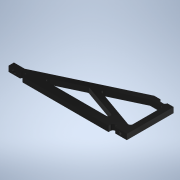
# Autodesk Inventor part: ForeArm_diagonal
Saved by Autodesk Inventor 2020.4 (Build 244396000, 396)
## iProperties
Created: 2016-05-04
Part Number: ForeArm_diagonal
Material: アセタール樹脂、黒
Document SubType Name: Modeling
Designer: hiroaki
Density: 1.425 g/cm^3
Appearance: 滑らか - 黒
Mass: 16.6114 g
Surface Area: 81.8888 cm^2
Volume: 11.6571 cm^3
Description: POM T5
Author: hiroaki
Autodesk Inventor part; units mm, degrees
ref_plane "YZ Plane" through (0, 0, 0) normal (1, 0, 0) x (0, 1, 0)
ref_plane "XZ Plane" through (0, 0, 0) normal (0, 1, 0) x (-1, 0, 0)
ref_plane "XY Plane" through (0, 0, 0) normal (0, 0, 1) x (1, 0, 0)
sketch "スケッチ1" plane through (0, 0, 0) normal (0, 0, 1) x (1, 0, 0)
  line L0 (-55, -21.75) -> (55, -21.75) construction
  line L1 (55, -21.75) -> (55, 21.75) construction
  line L2 (55, 21.75) -> (-55, 21.75) construction
  line L3 (-55, 21.75) -> (-55, -21.75) construction
  line L4 (-55, -21.75) -> (55, 21.75) construction
  line L5 (55, -21.75) -> (-55, 21.75) construction
  line L6 (-50, 21.75) -> (-50, -21.75) construction
  line L7 (0, 0) -> (0, 21.75) construction
  line L8 (0, 0) -> (-55, 0) construction
  line L9 (50, 21.75) -> (50, -11.2747) construction
  line L10 (-55, -21.75) -> (-44.2, -21.75)
  line L11 (47, 21.75) -> (47, 23.75)
  line L12 (47, 23.75) -> (45, 23.75)
  line L13 (45, 23.75) -> (45, 21.75)
  line L14 (49.2, 21.75) -> (55, 21.75)
  line L15 (55, 21.75) -> (55, -21.75)
  line L16 (55, -21.75) -> (44.2, -21.75)
  line L17 (-40, -21.75) -> (-40, -23.75)
  line L18 (-40, -23.75) -> (40, -23.75)
  line L19 (40, -23.75) -> (40, -21.75)
  arc A0 (42.8, 21.75) -> (47, 21.75) centre (44.9, 21.75) ccw
  arc A1 (45, 21.75) -> (49.2, 21.75) centre (47.1, 21.75) ccw
  arc A2 (-40, -21.75) -> (-44.2, -21.75) centre (-42.1, -21.75) ccw
  arc A3 (44.2, -21.75) -> (40, -21.75) centre (42.1, -21.75) ccw
  line L20 (-55, -21.75) -> (-55, -16.75)
  line L21 (42.8, 21.75) -> (37, 21.75)
  line L22 (49.45, 24.476) -> (52.55, 24.476) construction
  line L23 (52.55, 24.476) -> (52.55, 13.3235) construction
  line L24 (52.55, 13.3235) -> (49.45, 13.3235) construction
  line L25 (49.45, 13.3235) -> (49.45, 24.476) construction
  line L26 (51, 24.476) -> (51, 13.3235) construction
  line L27 (39.45, 24.476) -> (42.55, 24.476) construction
  line L28 (42.55, 24.476) -> (42.55, 13.9945) construction
  line L29 (42.55, 13.9945) -> (39.45, 13.9945) construction
  line L30 (39.45, 13.9945) -> (39.45, 24.476) construction
  line L31 (41, 24.476) -> (41, 13.9945) construction
  line L32 (-55, -16.75) -> (-45.4461, -16.75)
  line L33 (-44.5961, -16.5604) -> (37, 21.75)
  line L34 (39.7685, 17.5262) -> (10.0851, 3.5895) construction
  line L35 (-33.2353, -16.75) -> (50, -16.75) construction
  line L36 (50, -16.75) -> (50, 14.75) construction
  line L37 (48, 16.75) -> (38.5615, 16.75)
  line L38 (50, -16.75) -> (2.44, 0) construction
  line L39 (-1.5272, -1.8627) -> (-25.1196, -12.9396)
  line L40 (-0.0128, -1.7866) -> (31.439, -12.8636)
  line L41 (30.7746, -16.75) -> (-24.2696, -16.75)
  line L42 (10.2707, -0.1074) -> (47.3356, -13.1611)
  line L43 (50, -14.0995) -> (50, 16.75)
  arc A4 (47.3356, -13.1611) -> (50, -11.2747) centre (48, -11.2747) ccw
  arc A5 (10.0851, 3.5895) -> (10.2707, -0.1074) centre (10.9351, 1.7791) ccw
  line L44 (37.7115, 16.5604) -> (10.0851, 3.5895)
  arc A6 (38.5615, 16.75) -> (37.7115, 16.5604) centre (38.5615, 14.75) ccw
  arc A7 (50, 14.75) -> (48, 16.75) centre (48, 14.75) ccw
  arc A8 (-25.1196, -12.9396) -> (-24.2696, -16.75) centre (-24.2696, -14.75) ccw
  arc A9 (-0.0128, -1.7866) -> (-1.5272, -1.8627) centre (-0.6772, -3.6731) ccw
  arc A10 (30.7746, -16.75) -> (31.439, -12.8636) centre (30.7746, -14.75) ccw
  arc A11 (-45.4461, -16.75) -> (-44.5961, -16.5604) centre (-45.4461, -14.75) ccw
  point P0 (50, -21.75)
  point P1 (-45, -16.75)
  point P2 (38.1154, 16.75)
  point P3 (-0.7856, -1.5145)
  point P4 (42.4741, -16.75)
  point P5 (50, 14.75)
  point P6 (50, -11.2747)
  point P7 (46, 19.9611)
  dimension "d16" = 5
  dimension "d20" = 43.5
  dimension "d40" = 100
  dimension "d41" = 10
  dimension "d42" = 2.1
  dimension "d43" = 2
  dimension "d44" = 5
  dimension "d45" = 10
  dimension "d46" = 10
  dimension "d48" = 3.1
  dimension "d50" = 4
  dimension "d51" = -10
  dimension "d52" = 3.1
  dimension "d62" = 6
  dimension "d63" = 6
  dimension "d88" = 10
  dimension "d90" = 5
  dimension "d91" = 5
  dimension "d93" = 5
  dimension "d94" = 78.8236
  dimension "d96" = 39.4118
  dimension "d97" = 2.5
  dimension "d98" = 5
  dimension "d99" = 2
  dimension "d100" = 2
  dimension "d101" = 5
  dimension "d102" = 2
  dimension "d103" = 2
  dimension "d104" = 2
  dimension "d105" = 2
  constraints: 90 end point, 27 point on line, 24 point on circle, 19 tangent, 14 perpendicular, 12 centre point, 10 parallel, 8 collinear, 8 midpoint, 5 equal radius, 5 horizontal, 4 horizontal alignment, 2 symmetric about line, 2 vertical, 3 other
  measures "d16" distance between parallel lines of L3 L6
  measures "d20" distance of L2.end L0.start
  measures "d40" distance between parallel lines of L9 L6
  measures "d41" distance between parallel lines of L6 L17
  measures "d42" radius of A2
  measures "d43" distance between parallel lines of L0 L18
  measures "d44" distance from line of L10 L20.end
  measures "d45" distance between parallel lines of L1 L13
  measures "d46" distance from line of L21.end L11
  measures "d48" distance of L22.start L22.end
  measures "d50" distance between parallel lines of L1 L26
  measures "d51" distance between parallel lines of L26 L31
  measures "d52" distance of L27.start L27.end
  measures "d62" distance between parallel lines of L13 L26
  measures "d63" distance between parallel lines of L31 L11
  measures "d88" distance of L20.end point (-45, -16.75)
  measures "d90" distance between parallel lines of L33 L34
  measures "d91" distance between parallel lines of L1 L36
  measures "d93" distance between parallel lines of L16 L35
  measures "d94" distance of point (38.115, 16.75) L35.start
  measures "d96" distance of L38.end point (38.115, 16.75)
  measures "d97" distance between parallel lines of L40 L38
  measures "d98" distance between parallel lines of L40 L42
  measures "d99" radius of A4
  measures "d100" radius of A5
  measures "d101" distance between parallel lines of L37 L2
  measures "d102" radius of A6
  measures "d103" radius of A7
  measures "d104" radius of A8
  measures "d105" radius of A11
extrude "押し出し1" add sketch "スケッチ1" along normal blind 2.5 contours L20 L32 A11 L33 L21 A0 A1 L14 L15 L16 A3 L19 L18 L17 A2 L10
mirror "ミラー1" about plane through (0, -1, 0) normal (0, 0, -1) of "押し出し1"
sketch "スケッチ2" plane through (-55, -21.75, 2.5) normal (0, -1, 0) x (1, 0, 0)
  line L0 (0, -5) -> (0, 0)
  line L1 (15, -5) -> (95, -5) construction
  line L2 (55, -5) -> (55, 0) construction
  line L3 (15, 0) -> (95, 0) construction
  point P0 (55, -2.5)
  point P1 (103.6493, -2.5)
  point P2 (0, -2.5)
  constraints: 4 end point, 3 midpoint
hole "穴1" at (48.6493, -21.75, 0) direction (0, 1, 0) diameter 2.459 depth 2 thread size "M3x0.5" class "6H" standard "ISO Metric profile"
sketch "スケッチ4" plane through (49.2, 21.75, 2.5) normal (0, 1, 0) x (1, 0, 0)
  line L0 (5.8, 5) -> (5.8, 0) projected
  point P0 (-49.2, 2.5)
  point P1 (1.8, 2.5)
  point P2 (-8.2, 2.5)
  point P3 (5.8, 2.5)
  dimension "d53" = 4
  dimension "d54" = -10
  constraints: 2 horizontal alignment, 1 midpoint
  measures "d53" distance from line of point (1.8, 2.5) L0
  measures "d54" distance of point (-8.2, 2.5) point (1.8, 2.5)
hole "穴2" at (51, 21.75, 0) at (41, 21.75, 0) direction (0, -1, 0) diameter 2.459 depth 2.5 thread size "M3x0.5" class "6H" standard "ISO Metric profile"
sketch "スケッチ7" plane through (-55, -21.75, 2.5) normal (0, -1, 0) x (1, 0, 0)
  line L0 (0, -5) -> (0, 0) projected
  line L1 (15, 0) -> (95, 0) projected
  line L2 (15, -5) -> (95, -5) projected
  line L3 (0, -2.5) -> (5, -2.5)
  point P0 (55, -2.5)
  dimension "d80" = 5
  constraints: 2 end point, 1 horizontal, 1 midpoint
  measures "d80" distance from line of L3.end L0
hole "穴3" at (-50, -21.75, 0) direction (0, 1, 0) diameter 3 end through all
equation "\"d16\" = d4"
equation "\"d41\" = d3"
equation "\"d46\" = d45"
equation "\"d63\" = d62"
equation "\"d53\" = d50"
equation "\"d54\" = d51"
equation "\"d4\" = 5"
equation "\"d3\" = 10"
